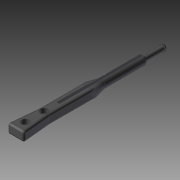
# Autodesk Inventor part: 6103C_Bulb Arm_CalibCoil
Saved by Autodesk Inventor 2021 (Build 250183000, 183)
## iProperties
Created: 2019-10-22
Part Number: 6103C_Bulb Arm_CalibCoil
Material: ABS Plastic
Document SubType Name: Modeling
Designer: RFLab
Density: 1.06 g/cm^3
Appearance: Smooth - White
Author: RFLab
Autodesk Inventor part; units mm, degrees
ref_plane "Work Plane3" through (0, 0, -39) normal (0, 0, -1) x (-1, 0, 0)
ref_plane "YZ Plane" through (0, 0, 0) normal (1, 0, 0) x (0, 1, 0)
sketch "Sketch8" plane through (0, 0, 0) normal (0, 0, 1) x (1, 0, 0)
  line L0 (-5.9, -5) -> (5.9, -5)
  line L1 (5.9, -5) -> (5.9, 5)
  line L2 (5.9, 5) -> (-5.9, 5)
  line L3 (-5.9, 5) -> (-5.9, -5)
  line L4 (-5.9, -5) -> (5.9, 5) construction
  line L5 (5.9, -5) -> (-5.9, 5) construction
  point P0 (0, 0)
  dimension "d41" = 11.8
  dimension "d42" = 10
  constraints: 12 end point, 2 midpoint, 2 parallel, 1 horizontal, 1 perpendicular
  measures "d41" distance of L2.end L1.end
  measures "d42" distance of L1.end L0.end
extrude "Extrusion8" add sketch "Sketch8" along normal blind 75
sketch "Sketch9" plane through (0, 0, 0) normal (0, 0, -1) x (-1, 0, 0)
  line L0 (5.9, 5) -> (5.9, -5) projected
  circle A0 centre (0, 0) radius 4.5
  line L1 (5.9, -5) -> (-5.9, -5) projected
  point P0 (0, 0)
  point P1 (5.9, 0)
  point P2 (0, -5)
  point P3 (5.9, 0)
  dimension "d45" = 9
  dimension "d134" = 11.8
  dimension "d135" = 10
  constraints: 3 midpoint, 2 horizontal alignment, 1 centre point, 1 vertical alignment
  measures "d45" diameter of A0
  measures "d134" distance of L0.end L1.end
  measures "d135" distance of L0.start L0.end
extrude "Extrusion9" add sketch "Sketch9" along normal blind 60
sketch "Sketch10" plane through (0, 0, 0) normal (0, 0, -1) x (-1, 0, 0)
  line L0 (5.9, -5) -> (-5.9, -5) projected
  line L1 (5.9, 5) -> (5.9, -5) projected
  line L2 (-5.9, 5) -> (5.9, 5) projected
  line L3 (-5.9, -5) -> (-5.9, 5) projected
ref_plane "Work Plane2" through (0, 0, -15) normal (0, 0, -1) x (-1, 0, 0)
sketch "Sketch11" plane through (0, 0, -15) normal (0, 0, -1) x (-1, 0, 0)
  circle A0 centre (0, 0) radius 4.5
  point P0 (0, 0)
  dimension "d140" = 9
  constraints: 1 centre point
  measures "d140" diameter of A0
loft "Loft3" add profiles "Sketch10", "Sketch11"
sketch "Sketch14" plane through (-5.9, 5, 75) normal (0, 1, 0) x (1, 0, 0)
  line L0 (11.8, 0) -> (0, 0) projected
  line L1 (0, 0) -> (11.8, 0) projected
  line L2 (5.9, 0) -> (5.9, 75)
  point P0 (5.9, 10)
  point P1 (5.9, 30)
  dimension "d64" = 10
  dimension "d65" = 30
  constraints: 2 end point, 2 point on line, 1 midpoint, 1 perpendicular
  measures "d64" distance from line of L0 point (5.9, 10)
  measures "d65" distance from line of L0 point (5.9, 30)
hole "Hole1" at (0, 5, 65) at (0, 5, 45) direction (0, -1, 0) diameter 4 end through all counterbore diameter 8 counterbore depth 5
sketch "Sketch15" plane through (-5.9, -5, 75) normal (0, -1, 0) x (1, 0, 0)
  circle A0 centre (5.9, -10) radius 2 projected
  circle A1 centre (5.9, -30) radius 2 projected
  line L0 (11.8, -75) -> (11.8, 0) projected
  line L1 (0, 0) -> (11.8, 0) projected
  line L2 (0, -75) -> (0, 0) projected
  line L3 (11.8, 0) -> (14.7, 0)
  line L4 (14.7, 0) -> (11.8, -30)
  line L5 (11.8, -75) -> (11.8, 0) projected
  line L6 (0, -75) -> (0, 0) projected
  line L7 (0, 0) -> (-2.9, 0)
  line L8 (-2.9, 0) -> (0, -30)
  line L9 (0, -75) -> (11.8, -75) projected
  point P0 (5.9, -75)
  dimension "d73" = 2.9
  dimension "d74" = 2.9
  constraints: 8 end point, 3 point on line, 2 horizontal alignment, 1 horizontal
  measures "d73" distance of L1.start L7.end
  measures "d74" distance of L0.end L3.end
extrude "Extrusion12" add sketch "Sketch15" against normal up to surface (10 mm away) contours L0 L3 L4 | L8 L7 L2
fillet "Fillet4" radius 2 12 edges at (-8.8, 0, 75) (8.8, 0, 75) (-7.35, 5, 60) (0, 5, 75) (7.35, 5, 60) (-5.9, 5, 22.5) (-5.9, -5, 22.5) (5.9, -5, 22.5) (7.35, -5, 60) (0, -5, 75) (5.9, 5, 22.5) (-7.35, -5, 60)
sketch "Sketch30" plane through (0, 0, -60) normal (0, 0, -1) x (-1, 0, 0)
  circle A0 centre (0, 0) radius 2.5
  dimension "d152" = 5
  constraints: 1 centre point, 1 coincident
  measures "d152" diameter of A0
extrude "Extrusion24" add sketch "Sketch30" along normal blind 20
sketch "Sketch31" plane through (0, 0, -80) normal (0, 0, -1) x (-1, 0, 0)
  circle A0 centre (0, 0) radius 2.5 projected
  circle A1 centre (0, 0) radius 3.5
  dimension "d155" = 1
  constraints: 1 centre point
  measures "d155" radial gap between concentric circles of A0 A1
extrude "Extrusion25" add sketch "Sketch31" along normal blind 2 contours A0 | A1
fillet "Fillet23" radius 2 1 edges at (3.5, 0, -82)
sketch "Sketch32" plane through (0, 5, 45) normal (0, 1, 0) x (1, 0, 0)
  line L0 (-2.5, 105) -> (2.5, 105) projected
  line L1 (-1.5, 15) -> (1.5, 15)
  line L2 (1.5, 15) -> (1.5, 105)
  line L3 (1.5, 105) -> (-1.5, 105)
  line L4 (-1.5, 105) -> (-1.5, 15)
  point P0 (0, 45)
  point P1 (-1.5, 105)
  dimension "d159" = 3
  dimension "d160" = 1.5
  dimension "d161" = 30
  constraints: 8 end point, 2 parallel, 1 horizontal, 1 perpendicular, 1 point on line
  measures "d159" distance between parallel lines of L4 L2
  measures "d160" distance from line of L4 point (0, 45)
  measures "d161" distance from line of point (0, 45) L1
extrude "Extrusion26" cut sketch "Sketch32" against normal up to surface round surface about axis through (0, 0, -60) along (0, 0, -1) radius 2.5 far side no
fillet "Fillet24" radius 2 1 edges at (0, -4.5, -60)
sketch "Sketch23" plane through (0, 0, -60) normal (0, 0, -1) x (-1, 0, 0)
  circle A0 centre (0, 0) radius 3.05
  circle A1 centre (0, 0) radius 4.5 projected
  line L0 (4.5, 0) -> (-4.5, 0)
  line L1 (1.5, -2.6557) -> (-1.5, -2.6557)
  line L2 (-1.5, -2.6557) -> (-1.5, -4.5)
  line L3 (-1.5, -4.5) -> (1.5, -4.5)
  line L4 (1.5, -4.5) -> (1.5, -2.6557)
  line L5 (0, 0) -> (-3.182, 3.182)
  line L6 (0, 0) -> (4.5, 0) construction
  line L7 (0, 0) -> (3.182, 3.182)
  line L8 (0, 0) -> (4.5, 0) construction
  point P0 (3.05, 0)
  point P1 (-3.05, 0)
  point P2 (0, -2.6557)
  point P3 (1.5, -4.2426)
  point P4 (-1.5, -4.2426)
  point P5 (-1.5, -2.6557)
  point P6 (2.1567, 2.1567)
  point P7 (-2.1567, 2.1567)
  dimension "d102" = 6.1
  dimension "d105" = 3
  dimension "d142" = 135
  dimension "d143" = 45
  dimension "d136" = 2
  dimension "d144" = 0.95
  constraints: 16 end point, 3 horizontal, 2 midpoint, 2 parallel, 1 perpendicular, 1 point on line
  measures "d136" distance of L1.start L1.end
  measures "d144" distance between parallel lines of L4 L1
sketch "Sketch26" plane through (3.05, 0, -64) normal (0, 1, 0) x (1, 0, 0)
  line L0 (0, -2) -> (0, 0) projected
  line L1 (-6.1, 0) -> (0, 0) projected
  line L2 (-6.1, -2) -> (-6.1, 0) projected
  line L3 (-1.3, -4) -> (-4.8, -4)
  line L4 (-4.8, -4) -> (-4.8, -2)
  line L5 (-4.8, -2) -> (-1.3, -2)
  line L6 (-1.3, -2) -> (-1.3, -4)
  line L7 (-6.1, -2) -> (0, -2) projected
  line L8 (1.45, -4) -> (-7.55, -4) projected
  point P0 (-3.05, -64)
  point P1 (-3.3025, -8)
  point P2 (-3.05, -2)
  dimension "d118" = 3.5
  constraints: 8 end point, 2 collinear, 2 midpoint, 2 parallel, 1 horizontal, 1 perpendicular
  measures "d118" distance between parallel lines of L6 L4
sketch "Sketch28" plane through (0, 0, -39) normal (0, 0, -1) x (-1, 0, 0)
  line L0 (4.25, 0) -> (5, 0) projected
  line L1 (-5, 0) -> (-4.25, 0) projected
  arc A0 (5, 0) -> (-5, 0) centre (0, 0) ccw projected
  arc A1 (2.2262, -3.6203) -> (4.25, 0) centre (0, 0) ccw projected
  line L2 (1.75, -4.4721) -> (1.75, -4.6837) projected
  arc A2 (2.2262, -3.6203) -> (1.75, -4.4721) centre (2.75, -4.4721) ccw projected
  arc A3 (-4.25, 0) -> (-2.2262, -3.6203) centre (0, 0) ccw projected
  arc A4 (-1.75, -4.4721) -> (-2.2262, -3.6203) centre (-2.75, -4.4721) ccw projected
  line L3 (-1.75, -4.4721) -> (-1.75, -4.6837) projected
  circle A5 centre (0, 0) radius 5
  line L4 (-1.75, 0) -> (-1.75, -4.6837) projected
  line L5 (-1.75, -4.4721) -> (-1.75, -4.6837)
  line L6 (1.75, 0) -> (1.75, -4.6837) projected
  line L7 (1.75, -4.4721) -> (1.75, -4.6837)
  arc A6 (-1.75, -4.6837) -> (1.75, -4.6837) centre (0, 0) ccw projected
  point P0 (0, 0)
  constraints: 4 end point, 2 collinear, 1 centre point, 1 coincident, 1 concentric
sketch "Sketch29" plane through (0, 0, -40) normal (0, 0, -1) x (-1, 0, 0)
  circle A0 centre (0, 0) radius 1.5
  dimension "d127" = 3
  constraints: 1 centre point, 1 coincident
  measures "d127" diameter of A0
equation "\"d74\" = d73"
body "Solid2"
